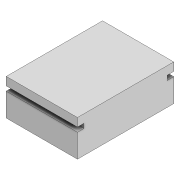
# Autodesk Inventor part: Placeholde_stepperdriverr
Saved by Autodesk Inventor 2022 (Build 260153000, 153)
## iProperties
Created: 2022-10-20
Part Number: Placeholde_stepperdriverr
Material: Generic
Document SubType Name: Modeling
Designer: MVeszpremi
Density: 1 g/cm^3
Appearance: Default
Author: MVeszpremi
Autodesk Inventor part; units mm, degrees
ref_plane "YZ Plane" through (0, 0, 0) normal (1, 0, 0) x (0, 1, 0)
ref_plane "XZ Plane" through (0, 0, 0) normal (0, 1, 0) x (-1, 0, 0)
ref_plane "XY Plane" through (0, 0, 0) normal (0, 0, 1) x (1, 0, 0)
sketch "Sketch1" plane through (0, 0, 0) normal (0, 1, 0) x (-1, 0, 0)
  line L0 (0, 0) -> (71, 0)
  line L1 (71, 0) -> (71, -96)
  line L2 (71, -96) -> (0, -96)
  line L3 (0, -96) -> (0, 0)
  dimension "d0" = 96
  dimension "d1" = 71
  constraints: 8 end point, 2 parallel, 1 horizontal, 1 perpendicular
  measures "d0" distance of L0.end L1.end
  measures "d1" distance of L1.end L2.end
extrude "Extrusion1" add sketch "Sketch1" along normal blind 36
sketch "Sketch2" plane through (0, 0, 0) normal (1, 0, 0) x (0, 0, -1)
  line L0 (96, 0) -> (0, 0) projected
  line L1 (0, 0) -> (0, 23.3)
  line L2 (0, 0) -> (0, 36) projected
  line L3 (96, 0) -> (96, 36) projected
  line L4 (0, 23.3) -> (96, 23.3)
  line L5 (96, 23.3) -> (96, 27.8)
  line L6 (96, 27.8) -> (0, 27.8)
  line L7 (0, 27.8) -> (0, 23.3)
  line L8 (6.5, 27.8) -> (89.5, 27.8)
  line L9 (89.5, 27.8) -> (89.5, 23.3)
  line L10 (89.5, 23.3) -> (6.5, 23.3)
  line L11 (6.5, 23.3) -> (6.5, 27.8)
  point P0 (6.5, 23.3)
  point P1 (0, 27.8)
  dimension "d4" = 23.3
  dimension "d5" = 4.5
  dimension "d6" = 83
  dimension "d7" = 6.5
  constraints: 18 end point, 4 parallel, 4 point on line, 2 horizontal, 2 perpendicular
  measures "d4" distance of L0.end L1.end
  measures "d5" distance of L1.end L6.end
  measures "d6" distance between parallel lines of L9 L11
  measures "d7" distance between parallel lines of L2 L11
extrude "Extrusion2" cut sketch "Sketch2" against normal blind 112.75 contours L4 L9 L6 L3 | L2 L6 L11 L4
body "Solid1"
